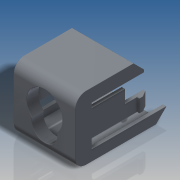
# Autodesk Inventor part: 99388-LtBluishGray
Saved by Autodesk Inventor 2016 SP2 (Build 200236200, 236)
## iProperties
Created: 2015-08-28
Part Number: 99388-LtBluishGray
Material: ABS Plastic
Document SubType Name: Modeling
Designer: D. Kohfeld
Density: 1.06 g/cm^3
Appearance: LtBluishGray
Mass: 2.51104 g
Surface Area: 41.332 cm^2
Volume: 2.36891 cm^3
Author: D. Kohfeld
Autodesk Inventor part; units mm, degrees
ref_plane "YZ Plane" through (0, 0, 0) normal (1, 0, 0) x (0, 1, 0)
ref_plane "XZ Plane" through (0, 0, 0) normal (0, 1, 0) x (-1, 0, 0)
ref_plane "XY Plane" through (0, 0, 0) normal (0, 0, 1) x (1, 0, 0)
sketch "Sketch2" plane through (0, 0, 0) normal (1, 0, 0) x (0, 1, 0)
  line L0 (-10.8, -21.6) -> (-10.8, 2)
  arc A0 (-7.2, 5.6) -> (-10.8, 2) centre (-7.2, 2) ccw
  line L1 (-7.2, 5.6) -> (7.2, 5.6)
  arc A1 (10.8, 2) -> (7.2, 5.6) centre (7.2, 2) ccw
  line L2 (10.8, 2) -> (10.8, -14)
  line L3 (10.8, -14) -> (7.2, -17.6)
  line L4 (7.2, -17.6) -> (6.4, -17.6)
  line L5 (6.4, -17.6) -> (6.4, 0)
  line L6 (6.4, 0) -> (4.8, 0)
  line L7 (4.8, 0) -> (4.8, -11.2)
  line L8 (4.8, -11.2) -> (0.4, -11.2)
  line L9 (0.4, -11.2) -> (0.4, -15.2)
  line L10 (0.4, -15.2) -> (-4, -15.2)
  line L11 (-4, -15.2) -> (-4, 0)
  line L12 (-4, 0) -> (-7.2, 0)
  line L13 (-7.2, 0) -> (-7.2, -25.2)
  line L14 (-7.2, -25.2) -> (-10.8, -21.6)
  line L15 (9.36, -15.44) -> (9.36, 4)
  line L16 (9.36, 4) -> (-9.6, 4)
  line L17 (-9.6, 4) -> (-9.6, -22.8)
  line L18 (-10.8, -10.8) -> (-9.6, -10.8)
  point P0 (0, 0)
  point P1 (0, 5.6)
  dimension "d0" = 21.6
  dimension "d1" = 3.6
  dimension "d2" = 30.8
  dimension "d3" = 5.6
  dimension "d4" = 45
  dimension "d5" = 3.6
  dimension "d6" = 4.4
  dimension "d7" = 4.4
  dimension "d8" = 4.4
  dimension "d9" = 0.8
  dimension "d10" = 23.2
  dimension "d11" = 1.6
  dimension "d12" = 16.8
  dimension "d13" = 20.8
  dimension "d14" = 1.44
  dimension "d15" = 1.2
  dimension "d16" = 1.6
  dimension "d21" = 14.4
  constraints: 38 end point, 9 vertical, 8 horizontal, 4 point on circle, 4 point on line, 4 tangent, 2 centre point, 2 horizontal alignment, 1 equal radius, 1 midpoint, 1 perpendicular, 1 vertical alignment
  measures "d0" distance between parallel lines of L2 L0
  measures "d1" radius of A1
  measures "d2" distance from line of L13.end L1
  measures "d3" distance between parallel lines of L12 L1
  measures "d4" angle of L13 L14
  measures "d5" distance between parallel lines of L0 L13
  measures "d6" distance between parallel lines of L7 L9
  measures "d7" distance between parallel lines of L11 L9
  measures "d8" distance between parallel lines of L5 L2
  measures "d9" distance of L3.end L4.end
  measures "d10" distance from line of L3.end L1
  measures "d11" distance between parallel lines of L5 L7
  measures "d12" distance between parallel lines of L8 L1
  measures "d13" distance between parallel lines of L10 L1
  measures "d14" distance between parallel lines of L2 L15
  measures "d15" distance between parallel lines of L0 L17
  measures "d16" distance between parallel lines of L1 L16
  measures "d21" distance from line of L13.end L18
extrude "Extrusion1" add sketch "Sketch2" along normal mid plane 20.8
extrude "Extrusion2" cut sketch "Sketch2" along normal mid plane 18.4 contours L17 L16 L15 L3 L4 L5 L6 L7 L8 L9 L10 L11 L12 L13 L14
extrude "Extrusion5" cut sketch "Sketch2" along normal mid plane 8 contours L0 L18 L17 L14
sketch "Sketch3" plane through (10.4, 0.4, -11.2) normal (0, 1, 0) x (1, 0, 0)
  line L0 (-1.2, 4) -> (0, 4) projected
  line L1 (-19.6, 0) -> (-19.6, 4) projected
  line L2 (-20.8, 4) -> (-19.6, 4) projected
  line L3 (-20.8, 0) -> (-20.8, 4) projected
  line L4 (-20.8, 0) -> (-19.6, 0) projected
  line L5 (-1.2, 4) -> (-1.2, 7.2)
  line L6 (-1.2, 7.2) -> (-0.4, 7.2)
  line L7 (-0.4, 7.2) -> (0.8, 5.2)
  line L8 (0.8, 4) -> (0, 4)
  line L9 (-19.6, 4) -> (-19.6, 7.2)
  line L10 (-19.6, 7.2) -> (-20.4, 7.2)
  line L11 (-20.4, 7.2) -> (-21.6, 5.2)
  line L12 (-21.6, 4) -> (-20.8, 4)
  line L13 (0.8, 5.2) -> (0.8, 4)
  line L14 (-21.6, 5.2) -> (-21.6, 4)
  point P0 (-10.4, -11.2)
  dimension "d32" = 3.2
  dimension "d33" = 0.8
  dimension "d34" = 1.2
  dimension "d35" = 0.8
  constraints: 20 end point, 4 equal length, 4 horizontal, 4 vertical
  measures "d32" distance between parallel lines of L12 L10
  measures "d33" distance of L12.start L2.start
  measures "d34" distance of L11.end L12.start
  measures "d35" distance of L9.end L10.end
extrude "Extrusion6" add sketch "Sketch3" against normal up to surface (4.4 mm away) contours L5 L6 L7 L13 L8 L0 | L2 L12 L14 L11 L10 L9
sketch "Sketch5" plane through (-10.4, -7.2, 5.6) normal (0, 0, 1) x (1, 0, 0)
  arc A0 (14.6012, 4.7163) -> (6.1988, 4.7163) centre (10.4, 9) ccw
  arc A1 (6.1988, 4.7163) -> (14.6012, 4.7163) centre (10.4, 3.8) ccw
  line L0 (0, 18) -> (20.8, 18) projected
  arc A2 (15.557, 3.9755) -> (5.243, 3.9755) centre (10.4, 9) ccw
  arc A3 (5.243, 3.9755) -> (15.557, 3.9755) centre (10.4, 3.8) ccw
  point P0 (10.4, 7.2)
  dimension "d51" = 12
  dimension "d52" = 8.6
  dimension "d53" = 5.2
  dimension "d54" = 3
  dimension "d55" = 14.4
  dimension "d56" = 10.32
  constraints: 8 point on circle, 4 centre point, 2 coincident, 2 vertical alignment
  measures "d51" diameter of A0
  measures "d52" diameter of A1
  measures "d53" distance of A0.centre A1.centre
  measures "d54" distance edge to line of A0 L0
  measures "d55" diameter of A2
  measures "d56" diameter of A3
extrude "Extrusion8" cut sketch "Sketch5" against normal through all contours A1 A0
sketch "Sketch6" plane through (9.2, -9.6, 4) normal (0, 0, -1) x (-1, 0, 0)
  arc A0 (4.9988, 7.1163) -> (13.4012, 7.1163) centre (9.2, 6.2) ccw projected
  arc A1 (13.4012, 7.1163) -> (4.9988, 7.1163) centre (9.2, 11.4) ccw projected
  arc A2 (14.357, 6.3755) -> (4.043, 6.3755) centre (9.2, 11.4) ccw projected
  arc A3 (4.043, 6.3755) -> (14.357, 6.3755) centre (9.2, 6.2) ccw projected
  point P0 (9.2, 9.6)
extrude "Extrusion9" add sketch "Sketch6" along normal blind 2.4
fillet "Fillet1" radius 0.1 110 edges at (-10.4, 10.8, -6) (-10.4, 0, 5.6) (-10.4, -9.7456, 4.5456) (-10.4, -10.8, -9.8) (-10.4, 9.7456, 4.5456) (10.4, 9.7456, 4.5456) (10.4, 0, 5.6) (10.4, -9.7456, 4.5456) (10.4, -10.8, -9.8) (10.4, 10.8, -6) (10.4, 6.4, -8.8) (10.4, 9, -15.8) (10.4, 6.8, -17.6) (10.4, 5.6, 0) (10.4, 4.8, -5.6) (10.4, 2.6, -11.2) (9.8, 4.8, -11.2) (9.2, 4.8, -5.6) (9.2, 5.6, 0) (9.2, 6.4, -8.8) (9.8, 6.4, -17.6) (9.8, 7.2, -17.6) (9.2, 6.8, -17.6) (9.2, 2.6, -11.2) (9.2, 0.4, -14.8) (10.4, 0.4, -13.2) (10.8, 0.4, -15.2) (11.2, -1.8, -15.2) (11.2, -1.8, -16.4) (11.2, 0.4, -15.8) (10.6, 0.4, -17.4) (9.6, 0.4, -18.4) (9.2, -1.8, -18.4) (10, -1.8, -18.4) (10.4, -4, -7.6) (10.8, -4, -15.2) (11.2, -4, -15.8) (10.6, -4, -17.4) (9.6, -4, -18.4) (9.2, -4, -9.2) (10.4, -5.6, 0) (9.2, -5.6, 0) (9.2, -7.2, -12.6) (10.4, -7.2, -12.6) (9.8, -7.2, -25.2) (10.4, -9, -23.4) (9.2, -8.4, -24) (6.6, -9.6, -22.8) (0, -9.6, -10.8) (-4, -9.6, -16.8) (-4, -10.8, -16.2) (0, -10.8, -10.8) (4, -9.6, -16.8) (4, -10.8, -16.2) (-4, -10.2, -22.2) (-6.6, -9.6, -22.8) (-9.2, -7.2, -12.6) (-10.4, -7.2, -12.6) (-9.2, -8.4, -24) (-9.8, -7.2, -25.2) (-10.4, -9, -23.4) (-9.2, -5.6, 0) (-10.4, -5.6, 0) (-9.2, -4, -9.2) (-10.4, -4, -7.6) (-11.2, -1.8, -15.2) (-10.8, -4, -15.2) (-11.2, -4, -15.8) (-10.6, -4, -17.4) (-9.2, -1.8, -18.4) (-9.6, -4, -18.4) (-10, -1.8, -18.4) (-9.6, 0.4, -18.4) (-10.6, 0.4, -17.4) (-11.2, -1.8, -16.4) (-11.2, 0.4, -15.8) (-10.4, 0.4, -13.2) (-9.2, 0.4, -14.8) (-9.2, 2.6, -11.2) (-10.4, 2.6, -11.2) (-9.8, 4.8, -11.2) (0, 9.36, -15.44) (0, 10.8, -14) (-9.2, 4.8, -5.6) (-10.4, 4.8, -5.6) (-9.2, 6.4, -8.8) (-9.2, 6.8, -17.6) (-9.8, 6.4, -17.6) (-10.4, 6.8, -17.6) (-9.8, 7.2, -17.6) (-9.2, 8.28, -16.52) (-10.4, 9, -15.8) (7.2, -10.8, -21.6) (4, -10.2, -22.2) (-7.2, -10.8, -21.6) (9.2, 8.28, -16.52) (-10.4, 5.6, 0) (-9.2, 5.6, 0) (-10.4, 6.4, -8.8) (-10.8, 0.4, -15.2) (0, 7.8, 5.5496) (5.9211, 2.7697, 5.6) (-5.9211, 2.7697, 5.6) (0, -7.7, 5.5651) (3.9004, -5.2101, 5.6) (-3.9004, -5.2101, 5.6) (0, 7.8, 1.6) (0, -7.7, 1.6) (0, -8.56, 1.6) (0, 9, 1.6)
equation "\"d11\" = wall"
equation "\"d16\" = wall"
equation "\"d30\" = lu"
equation "\"d36\" = lu"
equation "\"d50\" = lf"
equation "\"wall\" = 1.6"
equation "\"lu\" = 8"
equation "\"lf\" = 0.1"
body "Solid1"
